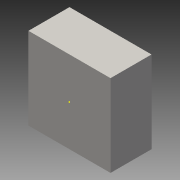
# Autodesk Inventor part: LED
Saved by Autodesk Inventor 2015 (Build 190159000, 159)
## iProperties
Created: 2016-01-03
Part Number: LED
Material: Generic
Document SubType Name: Modeling
Designer: david
Density: 1 g/cm^3
Appearance: Titanium
Mass: 0.032 g
Surface Area: 0.64 cm^2
Volume: 0.032 cm^3
Author: david
Autodesk Inventor part; units mm, degrees
ref_plane "YZ Plane" through (0, 0, 0) normal (1, 0, 0) x (0, 1, 0)
ref_plane "XZ Plane" through (0, 0, 0) normal (0, 1, 0) x (-1, 0, 0)
ref_plane "XY Plane" through (0, 0, 0) normal (0, 0, 1) x (1, 0, 0)
sketch "Sketch1" plane through (0, 0, 0) normal (0, 1, 0) x (-1, 0, 0)
  point P0 (0, 0)
sketch "Sketch2" plane through (0, 0, 0) normal (0, 1, 0) x (-1, 0, 0)
  line L0 (2, -2) -> (-2, -2)
  line L1 (-2, -2) -> (-2, 2)
  line L2 (-2, 2) -> (2, 2)
  line L3 (2, 2) -> (2, -2)
  line L4 (2, -2) -> (-2, 2) construction
  line L5 (-2, -2) -> (2, 2) construction
  point P0 (0, 0)
  dimension "d0" = 4
  dimension "d1" = 4
  constraints: 12 end point, 2 midpoint, 2 parallel, 1 horizontal, 1 perpendicular
  measures "d0" distance of L1.end L2.end
  measures "d1" distance of L0.end L1.end
extrude "Extrusion1" add sketch "Sketch2" along normal blind 2
body "Solid1"
